Autodesk Inventor part; units mm, degrees
(part 2 of 2)
  point P60 (53.634049, 45.855875)
  point P61 (45.855875, 53.634049)
  point P62 (60.422274, 52.6441)
  point P63 (49.249987, 57.028162)
  point P64 (57.028162, 49.249987)
  point P65 (53.139075, 53.139075)
  point P66 (32.003117, 62.890166)
  point P67 (21.840442, 67.099684)
  point P68 (35.676878, 71.75941)
  point P69 (23.677323, 71.534306)
  point P70 (33.839997, 67.324788)
  point P71 (28.75866, 69.429547)
  point P72 (5.5, 70.35)
  point P73 (-5.5, 70.35)
  point P74 (5.5, 79.95)
  point P75 (-5.5, 75.15)
  point P76 (5.5, 75.15)
  point P77 (0, 75.15)
  point P78 (-21.840442, 67.099684)
  point P79 (-32.003117, 62.890166)
  point P80 (-25.514203, 75.968928)
  point P81 (-33.839997, 67.324788)
  point P82 (-23.677323, 71.534306)
  point P83 (-28.75866, 69.429547)
  point P84 (-45.855875, 53.634049)
  point P85 (-53.634049, 45.855875)
  point P86 (-52.6441, 60.422274)
  point P87 (-57.028162, 49.249987)
  point P88 (-49.249987, 57.028162)
  point P89 (-53.139075, 53.139075)
  point P90 (-62.890166, 32.003117)
  point P91 (-67.099684, 21.840442)
  point P92 (-71.75941, 35.676878)
  point P93 (-71.534306, 23.677323)
  point P94 (-67.324788, 33.839997)
  point P95 (-69.429547, 28.75866)
  point P96 (-70.35, 5.5)
  point P97 (-70.35, -5.5)
  point P98 (-79.95, 5.5)
  point P99 (-75.15, -5.5)
  point P100 (-75.15, 5.5)
  point P101 (-75.15, 0)
  point P102 (-67.099684, -21.840442)
  point P103 (-62.890166, -32.003117)
  point P104 (-75.968928, -25.514203)
  point P105 (-67.324788, -33.839997)
  point P106 (-71.534306, -23.677323)
  point P107 (-69.429547, -28.75866)
  point P108 (-53.634049, -45.855875)
  point P109 (-45.855875, -53.634049)
  point P110 (-60.422274, -52.6441)
  point P111 (-49.249987, -57.028162)
  point P112 (-57.028162, -49.249987)
  point P113 (-53.139075, -53.139075)
  point P114 (-32.003117, -62.890166)
  point P115 (-21.840442, -67.099684)
  point P116 (-35.676878, -71.75941)
  point P117 (-23.677323, -71.534306)
  point P118 (-33.839997, -67.324788)
  point P119 (-28.75866, -69.429547)
  point P120 (-5.5, -26.35)
  point P121 (5.5, -26.35)
  point P122 (-5.5, -35.95)
  point P123 (5.5, -31.15)
  point P124 (-5.5, -31.15)
  point P125 (26.35, -5.5)
  point P126 (26.35, 5.5)
  point P127 (35.95, -5.5)
  point P128 (31.15, 5.5)
  point P129 (31.15, -5.5)
  point P130 (53.15, -5.5)
  point P131 (53.15, 5.5)
  point P132 (48.35, -5.5)
  point P133 (57.95, 5.5)
  point P134 (57.95, -5.5)
  point P135 (5.5, 26.35)
  point P136 (-5.5, 26.35)
  point P137 (5.5, 35.95)
  point P138 (-5.5, 31.15)
  point P139 (5.5, 31.15)
  point P140 (5.5, 53.15)
  point P141 (-5.5, 53.15)
  point P142 (5.5, 48.35)
  point P143 (-5.5, 57.95)
  point P144 (5.5, 57.95)
  point P145 (-26.35, 5.5)
  point P146 (-26.35, -5.5)
  point P147 (-35.95, 5.5)
  point P148 (-31.15, -5.5)
  point P149 (-31.15, 5.5)
  point P150 (-53.15, 5.5)
  point P151 (-53.15, -5.5)
  point P152 (-48.35, 5.5)
  point P153 (-57.95, -5.5)
  point P154 (-57.95, 5.5)
  dimension "d129" = 360
  dimension "d131" = 75.15
  dimension "d132" = 5.5
  dimension "d133" = 70.35
  dimension "d134" = 79.95
  dimension "d135" = 21.84044
  dimension "d136" = 23.67732
  dimension "d137" = 25.5142
  dimension "d138" = 28.75866
  dimension "d139" = 32.00312
  dimension "d140" = 33.84
  dimension "d141" = 67.09968
  dimension "d142" = 71.53431
  dimension "d143" = 75.96893
  dimension "d144" = 69.42955
  dimension "d145" = 62.89017
  dimension "d147" = 45.85587
  dimension "d148" = 49.24999
  dimension "d149" = 52.6441
  dimension "d150" = 53.13907
  dimension "d151" = 53.63405
  dimension "d152" = 57.02816
  dimension "d153" = 62.89017
  dimension "d154" = 53.63405
  dimension "d155" = 57.02816
  dimension "d156" = 60.42227
  dimension "d157" = 53.13907
  dimension "d158" = 45.85587
  dimension "d159" = 49.24999
  dimension "d160" = 32.00312
  dimension "d161" = 21.84044
  dimension "d162" = 33.84
  dimension "d163" = 28.75866
  dimension "d165" = 35.67688
  dimension "d166" = 67.09968
  dimension "d167" = 67.32479
  dimension "d168" = 69.42955
  dimension "d169" = 71.53431
  dimension "d170" = 71.75941
  dimension "d172" = 4.5
  dimension "d173" = 1.6
  dimension "d174" = 2.8
  dimension "d175" = 1.8
  dimension "d176" = 8.7
  dimension "d177" = 5
  dimension "d178" = 3
  dimension "d179" = 2.5
  dimension "d180" = 8.7
  dimension "d181" = 5
  dimension "d183" = 66.15
  dimension "d184" = 4.8
  dimension "d185" = 4.8
  dimension "d186" = 4.8
  dimension "d187" = 4.8
  dimension "d188" = 70.95
  dimension "d189" = 61.35
  dimension "d190" = 11
  dimension "d191" = 11
  dimension "d194" = 360
  dimension "d196" = 3
  constraints: 1524 end point, 148 point on line, 86 symmetric about line, 15 perpendicular, 4 coincident, 4 horizontal, 4 vertical, 3 point on circle, 2 collinear, 1 centre point, 1 midpoint, 1636 other
  measures "d131" distance of point (0, 0) L131.start
  measures "d132" distance of point (5.5, -75.15) L131.start
  measures "d133" vertical distance of point (5.5, -70.35) point (0, 0)
  measures "d134" vertical distance of point (0, 0) point (-5.5, -79.95)
  measures "d135" distance of point (21.84, 0) point (0, 0)
  measures "d136" distance of point (23.677, 0) point (0, 0)
  measures "d137" distance of point (0, 0) point (25.514, 0)
  measures "d138" distance of point (28.759, 0) point (0, 0)
  measures "d139" distance of point (32.003, 0) point (0, 0)
  measures "d140" distance of point (33.84, 0) point (0, 0)
  measures "d141" distance of point (21.84, -67.1) point (21.84, 0)
  measures "d142" distance of point (23.677, 0) point (23.677, -71.534)
  measures "d143" distance of point (25.514, -75.969) point (25.514, 0)
  measures "d144" distance of point (28.759, -69.43) point (28.759, 0)
  measures "d145" distance of point (32.003, 0) point (32.003, -62.89)
  measures "d147" distance of point (45.856, 0) point (0, 0)
  measures "d148" distance of point (49.25, 0) point (0, 0)
  measures "d149" distance of point (52.644, 0) point (0, 0)
  measures "d150" distance of point (53.139, 0) point (0, 0)
  measures "d151" distance of point (0, 0) point (53.634, 0)
  measures "d152" distance of point (57.028, 0) point (0, 0)
  measures "d153" distance of point (62.89, 0) point (0, 0)
  measures "d154" distance of point (45.856, 0) point (45.856, -53.634)
  measures "d155" distance of point (49.25, 0) point (49.25, -57.028)
  measures "d156" distance of point (52.644, 0) point (52.644, -60.422)
  measures "d157" distance of point (53.139, 0) point (53.139, -53.139)
  measures "d158" distance of point (53.634, -45.856) point (53.634, 0)
  measures "d159" distance of point (57.028, 0) point (57.028, -49.25)
  measures "d160" distance of point (62.89, 0) point (62.89, -32.003)
  measures "d161" distance of point (67.1, 0) point (67.1, -21.84)
  measures "d162" distance of point (67.325, 0) point (67.325, -33.84)
  measures "d163" distance of point (69.43, 0) point (69.43, -28.759)
  measures "d165" distance of point (71.759, 0) point (71.759, -35.677)
  measures "d166" distance of point (0, 0) point (67.1, 0)
  measures "d167" distance of point (0, 0) point (67.325, 0)
  measures "d168" distance of point (69.43, 0) point (0, 0)
  measures "d169" distance of point (0, 0) point (71.534, 0)
  measures "d170" distance of point (0, 0) point (71.759, 0)
  measures "d172" distance of L29.start L25.end
  measures "d173" distance of L29.start L27.end
  measures "d174" distance of L10.end L12.start
  measures "d175" distance of L13.start L12.start
  measures "d176" distance of L3.end L2.end
  measures "d177" distance of L1.end L2.end
  measures "d178" distance of L123.start L123.end
  measures "d179" distance of L123.end L124.end
  measures "d180" distance of L124.end L125.end
  measures "d181" distance of L125.end L126.end
  measures "d183" distance of point (0, 0) point (0, 66.15)
  measures "d184" distance of point (-5.5, -70.35) point (-5.5, -75.15)
  measures "d185" distance of point (-5.5, -79.95) point (-5.5, -75.15)
  measures "d186" distance of L129.start L129.end
  measures "d187" distance of L129.start L130.end
  measures "d188" vertical distance of L121.start point (5.5, 70.95)
  measures "d189" vertical distance of point (0, 0) point (5.5, 61.35)
  measures "d190" distance of L131.start L131.end
  measures "d191" distance of L173.start L534.end
  measures "d196" distance of L0.start L122.end
body "Solid2"
